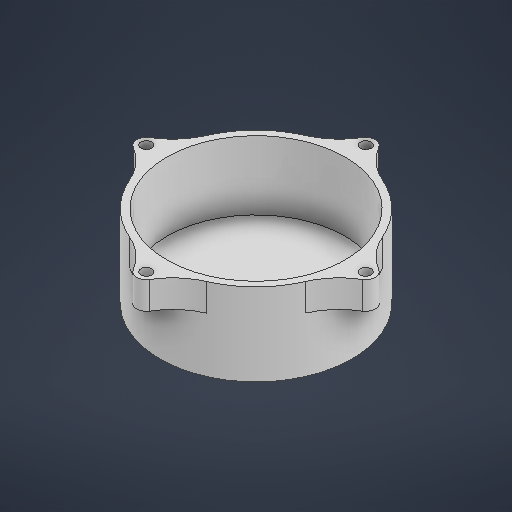
# Autodesk Inventor part: carcaza
Saved by Autodesk Inventor 2025.3 (Build 293356000, 356)
## iProperties
Created: 2025-10-20
Part Number: carcaza
Material: Generic
Document SubType Name: Modeling
Designer: sophi
Density: 1 g/cm^3
Appearance: Default
Author: sophi
Autodesk Inventor part; units mm, degrees
ref_plane "YZ Plane" through (0, 0, 0) normal (1, 0, 0) x (0, 1, 0)
sketch "Sketch1" plane through (0, 0, 0) normal (0, 1, 0) x (-1, 0, 0)
  circle A0 centre (0, 0) radius 35
  circle A1 centre (0, 0) radius 32.5
  dimension "d0" = 70
  dimension "d2" = 65
  constraints: 2 centre point, 1 coincident, 1 concentric
  measures "d0" diameter of A0
  measures "d2" diameter of A1
extrude "Extrusion3" add sketch "Sketch1" along normal blind 5 contours A1
extrude "Extrusion4" add sketch "Sketch1" along normal blind 30
ref_plane "Work Plane1" through (0, 17.5, 0) normal (0, 1, 0) x (-1, 0, 0)
ref_plane "Work Plane2" through (0, 0, -40) normal (0, 0, 1) x (1, 0, 0)
sketch "Sketch5" plane through (0, 30, 0) normal (0, 1, 0) x (1, 0, 0)
  circle A0 centre (-40, 0) radius 2
  circle A1 centre (-40, 0) radius 3.5
  circle A2 centre (0, 0) radius 35 projected
  arc A3 (-41.7894, 3.008) -> (-32.0691, 14.0204) centre (-54.0594, 23.6344) ccw
  arc A4 (-32.0691, -14.0204) -> (-41.7894, -3.008) centre (-54.0594, -23.6344) ccw
  circle A5 centre (0, -40) radius 3.5
  circle A6 centre (0, -40) radius 2
  arc A7 (-3.008, -41.7894) -> (-14.0204, -32.0691) centre (-23.6344, -54.0594) ccw
  arc A8 (14.0204, -32.0691) -> (3.008, -41.7894) centre (23.6344, -54.0594) ccw
  circle A9 centre (40, 0) radius 3.5
  circle A10 centre (40, 0) radius 2
  arc A11 (41.7894, -3.008) -> (32.0691, -14.0204) centre (54.0594, -23.6344) ccw
  arc A12 (32.0691, 14.0204) -> (41.7894, 3.008) centre (54.0594, 23.6344) ccw
  circle A13 centre (0, 40) radius 3.5
  circle A14 centre (0, 40) radius 2
  arc A15 (3.008, 41.7894) -> (14.0204, 32.0691) centre (23.6344, 54.0594) ccw
  arc A16 (-14.0204, 32.0691) -> (-3.008, 41.7894) centre (-23.6344, 54.0594) ccw
  point P0 (14.0204, -32.0691)
  point P1 (-14.0204, -32.0691)
  point P2 (32.0691, 14.0204)
  point P3 (-14.0204, 32.0691)
  point P4 (14.0204, 32.0691)
  dimension "d37" = 4
  dimension "d38" = 7
  dimension "d40" = 24
  dimension "d41" = 40
  dimension "d44" = 360
  constraints: 26 point on circle, 16 centre point, 4 coincident, 4 tangent, 1 equal radius, 1 horizontal alignment, 49 other
  measures "d37" diameter of A0
  measures "d38" diameter of A1
  measures "d40" radius of A3
  measures "d41" distance of point (0, 0) A0.centre
extrude "Extrusion9" add sketch "Sketch5" against normal blind 10 contours A1 | A1 A3 A2 A4 | A16 A13 A15 A2 | A2 A8 A5 A7 | A13 | A5 | A12 A9 A11 A2 | A9
body "Solid2"
